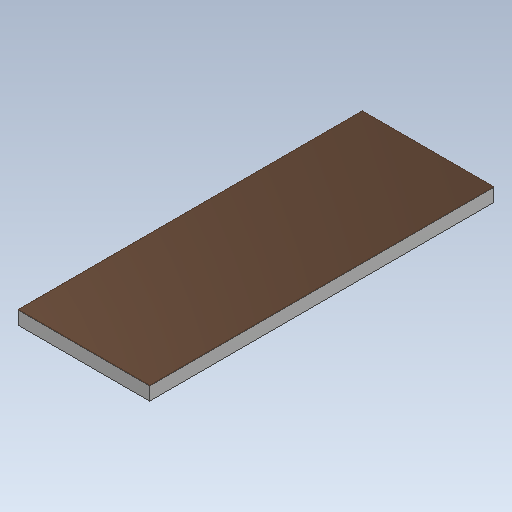
# Autodesk Inventor part: 071_0122_FoamKapton_long
Saved by Autodesk Inventor 2020 (Build 240168000, 168)
## iProperties
Created: 2020-04-29
Part Number: 071_0122_FoamKapton_long
Material: Generic
Document SubType Name: Modeling
Designer: deniz
Density: 1 g/cm^3
Appearance: Default
Author: deniz
Autodesk Inventor part; units mm, degrees
ref_plane "YZ Plane" through (0, 0, 0) normal (1, 0, 0) x (0, 1, 0)
ref_plane "XZ Plane" through (0, 0, 0) normal (0, 1, 0) x (-1, 0, 0)
ref_plane "XY Plane" through (0, 0, 0) normal (0, 0, 1) x (1, 0, 0)
sketch "Sketch1" plane through (0, 0, 0) normal (0, 1, 0) x (-1, 0, 0)
  line L0 (0, 0) -> (20, 0)
  line L1 (20, 0) -> (20, -52.4)
  line L2 (20, -52.4) -> (0, -52.4)
  line L3 (0, -52.4) -> (0, 0)
  dimension "d0" = 20
  dimension "d1" = 52.4
  constraints: 8 end point, 2 parallel, 1 horizontal, 1 perpendicular
  measures "d0" distance of L1.end L2.end
  measures "d1" distance of L0.end L1.end
extrude "Extrusion1" add sketch "Sketch1" against normal blind 2
extrude "Extrusion2" add sketch "Sketch1" along normal blind 0.1 separate body
equation "\"d1\" = d_bottom_length"
equation "\"d_bottom_length\" = 52.4"
